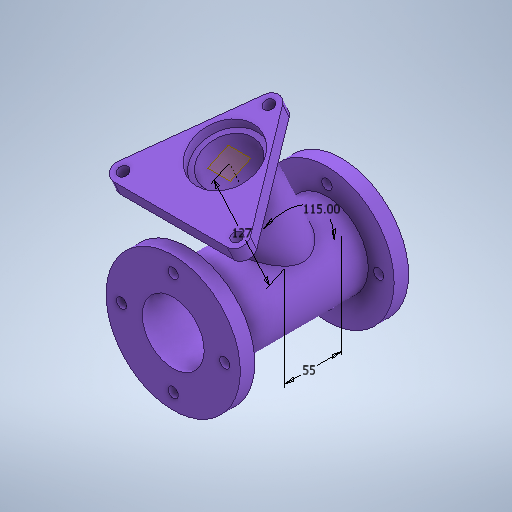
# Autodesk Inventor part: cad@63
Saved by Autodesk Inventor 2025.2 (Build 292293000, 293)
## iProperties
Created: 2025-04-21
Part Number: cad@63
Material: Generic
Document SubType Name: Modeling
Designer: spars
Density: 1 g/cm^3
Appearance: Violet
Author: spars
Autodesk Inventor part; units mm, degrees
ref_plane "YZ Plane" through (0, 0, 0) normal (1, 0, 0) x (0, 1, 0)
sketch "Sketch1" plane through (0, 0, 0) normal (0, 0, 1) x (1, 0, 0)
  circle A0 centre (0, 0) radius 40
  circle A1 centre (0, 0) radius 30
  dimension "d0" = 80
  dimension "d1" = 60
  constraints: 2 centre point, 2 coincident
  measures "d0" diameter of A0
  measures "d1" diameter of A1
extrude "Extrusion1" add sketch "Sketch1" along normal blind 135
sketch "Sketch2" plane through (0, 0, 135) normal (0, 0, 1) x (1, 0, 0)
  circle A0 centre (0, 0) radius 65
  circle A1 centre (0, 0) radius 30
  dimension "d4" = 130
  constraints: 2 centre point, 2 coincident
  measures "d4" diameter of A0
extrude "Extrusion2" add sketch "Sketch2" along normal blind 14
sketch "Sketch3" plane through (0, 0, 0) normal (0, 0, -1) x (-1, 0, 0)
  point P0 (0, 0)
sketch "Sketch4" plane through (0, 0, 149) normal (0, 0, 1) x (1, 0, 0)
  circle A0 centre (0, 0) radius 50
  circle A1 centre (-50, 0) radius 5
  circle A2 centre (0, -50) radius 5
  circle A3 centre (50, 0) radius 5
  circle A4 centre (0, 50) radius 5
  dimension "d7" = 100
  dimension "d8" = 10
  dimension "d11" = 360
  constraints: 4 centre point, 1 coincident, 1 horizontal alignment, 11 other
  measures "d8" diameter of A1
extrude "Extrusion3" cut sketch "Sketch4" against normal blind 14 contours A0 A3 | A0 A3 | A4 A0 | A0 A4 | A2 A0 | A0 A2 | A1 A0 | A0 A1
ref_plane "Work Plane1" through (0, 0, 67.5) normal (0, 0, 1) x (1, 0, 0)
mirror "Mirror1" about plane through (0, 0, 67.5) normal (0, 0, 1) of "Extrusion2", "Extrusion3"
ref_plane "Work Plane2" through (0, 0, 94) normal (0, 0, 1) x (1, 0, 0)
sketch "Sketch5" plane through (0, 0, 94) normal (0, 0, 1) x (1, 0, 0)
  circle A0 centre (0, 0) radius 30 projected
  line L0 (-30, 0) -> (30, 0)
  constraints: 2 end point, 2 point on circle, 1 horizontal
ref_plane "Work Plane3" through (-30, 0, 94) normal (0, -0.4226, 0.9063) x (1, 0, 0)
sketch "Sketch6" plane through (0, 0, 0) normal (1, 0, 0) x (0, 1, 0)
  point P0 (0, 0)
sketch "Sketch7" plane through (-30, 0, 94) normal (0, -0.4226, 0.9063) x (1, 0, 0)
  point P0 (30, -39.7261)
sketch "Sketch8" plane through (-30, 0, 94) normal (0, -0.4226, 0.9063) x (1, 0, 0)
  point P0 (30, -39.7261)
sketch "Sketch9" plane through (0, 0, 94) normal (0, 0, 1) x (1, 0, 0)
  point P0 (0, 0)
sketch "Sketch10" plane through (-30, 0, 94) normal (0, -0.4226, 0.9063) x (1, 0, 0)
  point P0 (30, -39.7261)
sketch "Sketch11" plane through (0, 0, 0) normal (1, 0, 0) x (0, 1, 0)
  line L0 (5, -14) -> (-5, -14) construction
  line L1 (0, -14) -> (0, 41) construction
  line L2 (0, 41) -> (115.1011, 94.6725) construction
  point P0 (0, 0)
  dimension "d18" = 127
  dimension "d19" = 115
  dimension "d20" = 55
  constraints: 4 end point, 1 midpoint, 1 vertical
  measures "d18" distance of L1.end L2.end
  measures "d19" angle of L1 L2
  measures "d20" distance of L1.start L1.end
ref_plane "Work Plane4" through (0, 115.1011, 94.6725) normal (0, 0.9063, 0.4226) x (-1, 0, 0)
sketch "Sketch12" plane through (0, 115.1011, 94.6725) normal (0, 0.9063, 0.4226) x (-1, 0, 0)
  circle A0 centre (0, 0) radius 30
  circle A1 centre (0, 0) radius 25
  point P0 (0, -37.1586)
  dimension "d21" = 60
  dimension "d22" = 50
  constraints: 2 centre point, 1 coincident
  measures "d21" diameter of A0
  measures "d22" diameter of A1
extrude "Extrusion4" add sketch "Sketch12" against normal up to next
sketch "Sketch13" plane through (0, 115.1011, 94.6725) normal (0, 0.9063, 0.4226) x (1, 0, 0)
  line L0 (54.3855, -57.451) -> (-55.6145, -57.451)
  line L1 (-64.2747, -42.451) -> (-9.2747, 52.8118)
  line L2 (8.0458, 52.8118) -> (63.0458, -42.451)
  arc A0 (54.3855, -57.451) -> (63.0458, -42.451) centre (54.3855, -47.451) ccw
  arc A1 (-64.2747, -42.451) -> (-55.6145, -57.451) centre (-55.6145, -47.451) ccw
  arc A2 (8.0458, 52.8118) -> (-9.2747, 52.8118) centre (-0.6145, 47.8118) ccw
  line L3 (54.3855, -47.451) -> (-55.6145, -47.451) construction
  circle A3 centre (54.3855, -47.451) radius 5
  circle A4 centre (-55.6145, -47.451) radius 5
  circle A5 centre (-0.6145, 47.8118) radius 5
  line L4 (-0.6145, -57.451) -> (-0.6145, -2.451) construction
  point P0 (0, 37.1586)
  dimension "d25" = 10
  dimension "d26" = 110
  dimension "d28" = 10
  dimension "d29" = 10
  dimension "d30" = 10
  dimension "d31" = 55
  constraints: 10 end point, 6 centre point, 6 point on circle, 6 tangent, 3 coincident, 2 equal length, 2 equal radius, 2 horizontal, 1 midpoint, 1 vertical
  measures "d25" radius of A0
  measures "d26" distance of L3.start L3.end
  measures "d28" diameter of A3
  measures "d29" diameter of A4
  measures "d30" diameter of A5
  measures "d31" distance of L4.start L4.end
extrude "Extrusion5" add sketch "Sketch13" along normal blind 10 and the other way blind 5
sketch "Sketch14" plane through (0, 124.1642, 98.8987) normal (0, 0.9063, 0.4226) x (1, 0, 0)
  circle A0 centre (0, 0) radius 25 projected
  circle A1 centre (0, 0) radius 30
  point P0 (0, 37.1586)
  constraints: 1 centre point, 1 coincident
extrude "Extrusion6" cut sketch "Sketch14" against normal blind 10 contours A0 | A1
sketch "Sketch15" plane through (0, 115.1011, 94.6725) normal (0, 0.9063, 0.4226) x (1, 0, 0)
  circle A0 centre (0, 0) radius 30 projected
  circle A1 centre (0, 0) radius 25
  point P0 (0, 37.1586)
  dimension "d38" = 50
  constraints: 1 centre point, 1 coincident
  measures "d38" diameter of A1
extrude "Extrusion7" cut sketch "Sketch15" against normal blind 120 contours A1
body "Solid1"
